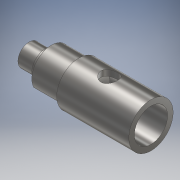
# Autodesk Inventor part: drive shaft
Saved by Autodesk Inventor 2017 (Build 210142000, 142)
## iProperties
Created: 2018-08-02
Part Number: drive shaft
Material: Stainless Steel
Document SubType Name: Modeling
Designer: jakub.tomczynski
Density: 8 g/cm^3
Appearance: Semi-Polished
Author: jakub.tomczynski
Autodesk Inventor part; units mm, degrees
ref_plane "YZ Plane" through (0, 0, 0) normal (1, 0, 0) x (0, 1, 0)
ref_plane "XZ Plane" through (0, 0, 0) normal (0, 1, 0) x (-1, 0, 0)
sketch "Sketch1" plane through (0, 0, 0) normal (0, 0, 1) x (1, 0, 0)
  line L0 (0, 0) -> (-11, 0)
  line L1 (-11, 0) -> (-11, 1)
  line L2 (-11, 1) -> (-9.5, 1)
  line L3 (-9.5, 1) -> (-9.5, 1.25)
  line L4 (-9.5, 1.25) -> (-9, 1.25)
  line L5 (-9, 1.25) -> (-9, 1.75)
  line L6 (-9, 1.75) -> (-6.5, 1.75)
  line L7 (-6.5, 1.75) -> (-6.5, 2)
  line L8 (-6.5, 2) -> (0, 2)
  line L9 (0, 2) -> (0, 0)
  dimension "d1" = 4
  dimension "d2" = 2
  dimension "d3" = 2.5
  dimension "d4" = 3.5
  dimension "d7" = 2.5
  dimension "d8" = 0.5
  dimension "d9" = 1.5
  dimension "d23" = 6.5
  constraints: 20 end point, 8 perpendicular, 1 horizontal, 1 vertical
  measures "d1" diameter of L8 L0
  measures "d2" diameter of L2 L0
  measures "d3" diameter of L4 L0
  measures "d4" diameter of L6 L0
  measures "d7" distance between parallel lines of L7 L5
  measures "d8" distance between parallel lines of L5 L3
  measures "d9" distance between parallel lines of L3 L1
  measures "d23" distance between parallel lines of L9 L7
revolve "Revolution1" add sketch "Sketch1" angle 360 about axis through (0, 0, 0) along (-1, 0, 0)
hole "motor shaft" at (0, 0, 0) direction (-1, 0, 0) diameter 3 depth 5.2 tip angle 118
sketch "Sketch2" plane through (-11, 0, 0) normal (-1, 0, 0) x (0, 0, 1)
  circle A0 centre (0, 0) radius 2 projected
  line L0 (-0.75, -1.854) -> (-0.75, 1.854)
  dimension "d11" = 0.75
  constraints: 2 end point, 2 point on circle, 1 vertical
  measures "d11" distance from line of point (0, 0) L0
extrude "D" cut sketch "Sketch2" against normal up to surface (4.5 mm away) contours L0 A0 picked at (-1.1667, 0)
ref_plane "Work Plane1" through (-3.25, 0, -2) normal (0, 0, 1) x (1, 0, 0)
sketch "Sketch3" plane through (-3.25, 0, -2) normal (0, 0, 1) x (1, 0, 0)
  point P0 (3.25, 0)
  point P1 (-0.5, 0)
  dimension "d14" = 3.75
  constraints: 1 horizontal alignment
  measures "d14" distance of point (3.25, 0) point (-0.5, 0)
hole "Hole1" at (-3.75, 0, -2) direction (0, 0, 1) diameter 1.5 end through all
body "Solid1"
